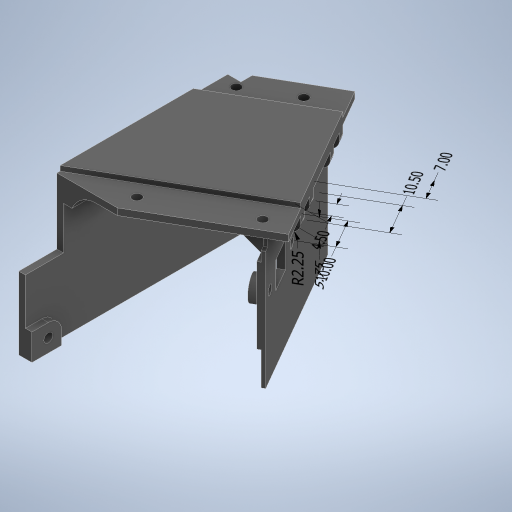
# Autodesk Inventor part: flame_side_right
Saved by Autodesk Inventor 2024.1 (Build 281209000, 209)
## iProperties
Created: 2025-03-06
Part Number: flame_side_right
Material: 一般
Document SubType Name: Modeling
Designer: hibik
Density: 1 g/cm^3
Appearance: 既定
Author: hibik
Autodesk Inventor part; units mm, degrees
ref_plane "YZ Plane" through (0, 0, 0) normal (1, 0, 0) x (0, 1, 0)
ref_plane "XZ Plane" through (0, 0, 0) normal (0, 1, 0) x (-1, 0, 0)
ref_plane "XY Plane" through (0, 0, 0) normal (0, 0, 1) x (1, 0, 0)
sketch "スケッチ1" plane through (0, 0, 0) normal (0, 1, 0) x (-1, 0, 0)
  line L0 (0, 0) -> (-75, 129.9038)
  line L1 (0, 0) -> (9.1573, 5.287) construction
  line L2 (-46.25, 80.1073) -> (0, 106.8098)
  line L3 (-28.75, 49.7965) -> (0, 66.3953)
  line L4 (-37.5, 64.9519) -> (-18.3005, 76.0367) construction
  line L5 (25.9887, 0) -> (-91.8315, 0) projected
  line L6 (0, 0) -> (0, 106.8098)
  line L7 (-51.25, 88.7676) -> (0, 118.3568)
  line L8 (0, 118.3568) -> (0, 106.8098)
  line L9 (-23.75, 41.1362) -> (0, 54.8483)
  dimension "d0" = 150
  dimension "d1" = 60
  dimension "d2" = 57.5
  dimension "d5" = 10
  constraints: 18 end point, 6 point on line, 4 perpendicular, 2 vertical, 1 midpoint, 1 parallel, 2 other
  measures "d0" distance from line of L0.end L1
  measures "d1" angle of L0 L5
  measures "d2" distance between parallel lines of L1 L3
  measures "d5" distance between parallel lines of L3 L9
extrude "押し出し1" add sketch "スケッチ1" along normal blind 1.5 contours L0 L2 L6 L3
extrude "押し出し2" add sketch "スケッチ1" against normal blind 2 contours L0 L3 L6 L9 | L0 L2 L6 L3 | L0 L7 L8 L2
sketch "スケッチ2" plane through (0, 1.5, 66.3953) normal (-1, 0, 0) x (0, 0, 1)
  line L0 (-22.0385, -1.5) -> (52.9615, -1.5)
  line L1 (52.9615, -1.5) -> (52.9615, -43.5)
  line L2 (52.9615, -43.5) -> (-22.0385, -43.5)
  line L3 (-22.0385, -43.5) -> (-22.0385, -1.5)
  line L4 (40.4145, -1.5) -> (51.9615, -1.5) projected
  line L5 (-22.0385, -11.5) -> (52.9615, -11.5)
  line L6 (51.9615, -3.5) -> (-11.547, -3.5) projected
  line L7 (51.9615, -1.5) -> (51.9615, -3.5) projected
  point P0 (-66.3953, -1.5)
  point P1 (20.2073, -3.5)
  point P2 (15.4615, -11.5)
  dimension "d8" = 75
  dimension "d9" = 32
  dimension "d12" = 10
  dimension "d23" = 1
  constraints: 10 end point, 2 midpoint, 2 parallel, 2 perpendicular, 2 point on line, 1 collinear, 1 horizontal
  measures "d8" distance of L0.start L0.end
  measures "d9" distance between parallel lines of L2 L5
  measures "d12" distance between parallel lines of L0 L5
  measures "d23" distance between parallel lines of L7 L1
extrude "押し出し3" add sketch "スケッチ2" against normal blind 2
sketch "スケッチ3" plane through (2, 1.5, 66.3953) normal (1, 0, 0) x (0, 0, -1)
  circle A0 centre (-47.9615, -12.5) radius 4
  circle A1 centre (17.0385, -12.5) radius 4
  line L0 (-52.9615, -43.5) -> (22.0385, -43.5) projected
  line L1 (-52.9615, -8.5) -> (22.0385, -8.5)
  line L2 (22.0385, -43.5) -> (22.0385, -1.5) projected
  line L3 (-51.9615, -8.5) -> (-51.9615, -18.5112) construction
  line L4 (-52.9615, -8.5) -> (-43.9615, -8.5)
  line L5 (-43.9615, -8.5) -> (-43.9615, -16.5)
  line L6 (-43.9615, -16.5) -> (-52.9615, -16.5)
  line L7 (-52.9615, -16.5) -> (-52.9615, -8.5)
  line L8 (22.0385, -8.5) -> (13.0385, -8.5)
  line L9 (13.0385, -8.5) -> (13.0385, -16.5)
  line L10 (13.0385, -16.5) -> (22.0385, -16.5)
  line L11 (22.0385, -16.5) -> (22.0385, -8.5)
  line L12 (22.0385, -1.5) -> (0, -1.5) projected
  line L13 (0, 0) -> (-40.4145, 0) projected
  line L14 (-40.4145, -1.5) -> (0, -1.5) projected
  line L15 (-40.4145, -1.5) -> (-40.4145, 0) projected
  line L16 (0, -1.5) -> (0, 0) projected
  line L17 (-40.4145, -1.5) -> (0, -1.5)
  line L18 (-52.9615, -1.5) -> (-52.9615, -43.5) projected
  line L19 (-40.4145, -1.5) -> (-52.9615, -1.5) projected
  line L20 (-52.9615, -35.5) -> (22.0385, -35.5)
  circle A2 centre (-47.9615, -39.5) radius 4
  circle A3 centre (17.0385, -39.5) radius 4
  line L21 (-43.9615, -39.5) -> (-43.9615, -43.5)
  line L22 (13.0385, -39.5) -> (13.0385, -43.5)
  point P0 (66.3953, -1.5)
  point P1 (13.0385, -12.5)
  point P2 (17.0385, -16.5)
  point P3 (22.0385, -16.5)
  point P4 (-47.9615, -16.5)
  point P5 (-43.9615, -12.5)
  point P6 (-47.9615, -8.5)
  point P7 (-47.9615, -35.5)
  point P8 (17.0385, -35.5)
  dimension "d13" = 8
  dimension "d14" = 35
  dimension "d15" = 65
  dimension "d24" = 1
  constraints: 28 end point, 7 horizontal, 7 tangent, 6 point on line, 5 perpendicular, 4 parallel, 3 vertical, 2 centre point, 2 vertical alignment, 1 collinear, 1 equal radius, 7 other
  measures "d13" diameter of A0
  measures "d14" distance between parallel lines of L0 L1
  measures "d15" distance of A1.centre A0.centre
  measures "d24" distance between parallel lines of L18 L3
extrude "押し出し4" add sketch "スケッチ3" along normal blind 2 contours A0 | A0 L1 L5 | A0 L6 L7 L1 | L1 L18 L19 L14 L12 L2 | L1 A1 L9 | L20 A2 L0 L18 | L1 L2 L10 A1 | A1 | A2 | A2 L21 L0 | L20 L2 L0 A3 | A3 | A3 L0 L22
sketch "スケッチ4" plane through (4, 1.5, 66.3953) normal (1, 0, 0) x (0, 0, -1)
  arc A0 (-47.9615, -16.5) -> (-43.9615, -12.5) centre (-47.9615, -12.5) ccw projected
  arc A1 (13.0385, -12.5) -> (17.0385, -16.5) centre (17.0385, -12.5) ccw projected
  circle A2 centre (-47.9615, -12.5) radius 1.35
  circle A3 centre (17.0385, -12.5) radius 1.35
  circle A4 centre (17.0385, -39.5) radius 1.35
  circle A5 centre (-47.9615, -39.5) radius 1.35
  arc A6 (17.0385, -35.5) -> (13.0385, -39.5) centre (17.0385, -39.5) ccw projected
  arc A7 (-43.9615, -39.5) -> (-47.9615, -35.5) centre (-47.9615, -39.5) ccw projected
  point P0 (66.3953, -1.5)
  dimension "d19" = 2.7
  dimension "d20" = 2.7
  constraints: 4 centre point, 2 coincident, 2 concentric, 2 equal radius
  measures "d19" diameter of A2
  measures "d20" diameter of A3
extrude "押し出し5" cut sketch "スケッチ4" against normal through all
sketch "スケッチ5" plane through (0, -2, 0) normal (0, -1, 0) x (1, 0, 0)
  line L0 (31.6173, 108.7628) -> (-5, 108.7628) construction
  line L1 (51.25, 88.7676) -> (4, 116.0474) projected
  line L2 (0, 44.3568) -> (0, 119.3568) projected
  line L3 (18.3494, 107.7628) -> (0, 107.7628)
  line L4 (4, 116.0474) -> (4, 119.3568) projected
  line L5 (0, 119.3568) -> (4, 119.3568) projected
  point P0 (0, 0)
  point P1 (0, 106.8098)
  dimension "d25" = 1
  constraints: 2 end point, 2 point on line, 1 parallel
  measures "d25" distance between parallel lines of L0 L3
extrude "押し出し6" cut sketch "スケッチ5" along normal mid plane 10
fillet "フィレット1" radius 8 1 edges at (4, -2, 80.1508)
sketch "スケッチ6" plane through (0, 0, 0) normal (0, 1, 0) x (1, 0, 0)
  circle A0 centre (17.5897, -50.4663) radius 1.6 construction
  circle A1 centre (4.5994, -57.9663) radius 1.6 construction
  circle A2 centre (43.3666, -88.7131) radius 1.6 construction
  circle A3 centre (18.4391, -101.9375) radius 1.6 construction
  circle A4 centre (17.5897, -50.4663) radius 1.35
  circle A5 centre (4.5994, -57.9663) radius 1.35
  circle A6 centre (18.4391, -101.9375) radius 1.35
  circle A7 centre (43.3666, -88.7131) radius 1.35
  point P0 (0, 0)
  dimension "d29" = 2.7
  constraints: 4 centre point, 4 coincident, 3 equal radius
  measures "d29" diameter of A4
extrude "押し出し7" cut sketch "スケッチ6" against normal through all
ref_plane "作業平面2" through (3.75, 0, 72.8905) normal (-0.5, 0, -0.8660254) x (-0.8660254, 0, 0.5)
ref_plane "作業平面1" through (8.75, 0, 81.5507) normal (-0.5, 0, -0.8660254) x (-0.8660254, 0, 0.5)
sketch "スケッチ7" plane through (3.75, 0, 72.8905) normal (-0.5, 0, -0.8660254) x (-0.8660254, 0, 0.5)
  circle A0 centre (-30.9476, -4.25) radius 2.25
  circle A1 centre (-30.9476, -4.25) radius 1
  line L0 (-33.1976, -2) -> (4.7927, -2) projected
  line L1 (-33.1976, 0) -> (-33.1976, -2) projected
  line L2 (-33.1976, -2) -> (-33.1976, -4.25)
  line L3 (-28.6976, -4.25) -> (-28.6976, -2)
  point P0 (-30.9476, -2)
  dimension "d33" = 2
  dimension "d34" = 4.5
  constraints: 4 end point, 3 tangent, 2 centre point, 2 point on circle, 1 coincident, 1 parallel, 1 point on line, 1 vertical
  measures "d33" diameter of A1
  measures "d34" diameter of A0
extrude "押し出し8" add sketch "スケッチ7" against normal blind 3
sketch "スケッチ8" plane through (0, 0, 66.3953) normal (-0.5, 0, -0.8660254) x (-0.8660254, 0, 0.5)
  arc A0 (-33.1976, -4.25) -> (-28.6976, -4.25) centre (-30.9476, -4.25) ccw projected
  circle A1 centre (-30.9476, -4.25) radius 1 projected
  line L0 (-28.6976, -4.25) -> (-28.6976, -2) projected
  line L1 (-33.1976, -2) -> (-28.6976, -2) projected
  line L2 (-33.1976, -2) -> (-33.1976, -4.25) projected
  point P0 (-33.1976, 0)
extrude "押し出し9" add sketch "スケッチ8" against normal blind 3
mirror "ミラー1" about plane through (8.75, 0, 81.5507) normal (-0.5, 0, -0.8660254) of "押し出し9", "押し出し8"
sketch "スケッチ9" plane through (0, 1.5, 66.3953) normal (-1, 0, 0) x (0, 0, 1)
  line L0 (-22.0385, -8.5) -> (-10.4445, -8.5)
  line L1 (-10.4445, -8.5) -> (-10.4445, -21.5)
  line L2 (-10.4445, -21.5) -> (-22.0385, -21.5)
  line L3 (-22.0385, -21.5) -> (-22.0385, -8.5)
  line L4 (41.3675, -8.5) -> (52.9615, -8.5)
  line L5 (52.9615, -8.5) -> (52.9615, -21.5)
  line L6 (52.9615, -21.5) -> (41.3675, -21.5)
  line L7 (41.3675, -21.5) -> (41.3675, -8.5)
  line L8 (52.9615, -43.5) -> (52.9615, -8.5) projected
  line L9 (52.9615, -8.5) -> (41.3675, -8.5) projected
  line L10 (-22.0385, -1.5) -> (-22.0385, -43.5) projected
  line L11 (41.3675, -8.5) -> (41.3675, -1.5) projected
  line L12 (-10.4445, -8.5) -> (-10.4445, -1.5)
  line L13 (-22.0385, -1.5) -> (0, -1.5) projected
  point P0 (-66.3953, -1.5)
  dimension "d60" = 0
  dimension "d63" = 13
  constraints: 18 end point, 4 parallel, 3 collinear, 2 equal length, 2 horizontal, 2 perpendicular, 2 point on line, 1 vertical
  measures "d60" distance between parallel lines of L9 L4
  measures "d63" distance between parallel lines of L6 L4
extrude "押し出し10" cut sketch "スケッチ9" against normal up to surface (4 mm away)
sketch "スケッチ10" plane through (0, -2, 0) normal (0, -1, 0) x (1, 0, 0)
  line L0 (4, 55.9508) -> (0, 55.9508) projected
  line L1 (0, 55.9508) -> (0, 66.3953) projected
  line L2 (28.75, 49.7965) -> (0, 66.3953) projected
  line L3 (28.75, 49.7965) -> (23.75, 41.1362) projected
  line L4 (23.75, 41.1362) -> (4, 52.5389) projected
  line L5 (4, 52.5389) -> (4, 55.9508) projected
  circle A0 centre (4.5994, 57.9663) radius 1.35 projected
  circle A1 centre (17.5897, 50.4663) radius 1.35 projected
  line L6 (0, 44.3568) -> (0, 119.3568) projected
  line L7 (0, 44.3568) -> (4, 44.3568) projected
  line L8 (4, 53.3568) -> (4, 44.3568) projected
  line L9 (2, 53.3568) -> (4, 53.3568) projected
  line L10 (2, 110.3568) -> (2, 53.3568) projected
  line L11 (2, 110.3568) -> (4, 110.3568) projected
  line L12 (4, 119.3568) -> (4, 110.3568) projected
  line L13 (0, 119.3568) -> (4, 119.3568) projected
  line L14 (4, 55.9508) -> (18.0903, 55.9508)
  point P0 (0, 0)
  constraints: 2 end point, 1 horizontal, 1 point on line
extrude "押し出し11" cut sketch "スケッチ10" along normal through all contours L14 L2 L3 L4 L5
sketch "スケッチ11" plane through (0, -2, 0) normal (0, -1, 0) x (1, 0, 0)
  line L0 (46.0538, 91.7676) -> (18.5538, 44.1362)
  line L1 (18.5538, 44.1362) -> (16.8218, 45.1362)
  line L2 (16.8218, 45.1362) -> (44.3218, 92.7676)
  line L3 (44.3218, 92.7676) -> (46.0538, 91.7676)
  line L4 (34, 58.8897) -> (41, 71.0141) projected
  line L5 (51.25, 88.7676) -> (18.3494, 107.7628) projected
  line L6 (4, 52.5389) -> (23.75, 41.1362) projected
  point P0 (0, 0)
  dimension "d66" = 2
  dimension "d68" = 6
  constraints: 8 end point, 3 parallel, 2 collinear, 1 perpendicular
  measures "d66" distance between parallel lines of L2 L0
  measures "d68" distance between parallel lines of L4 L0
extrude "押し出し12" add sketch "スケッチ11" along normal blind 22
sketch "スケッチ14" plane through (16.8218, -24, 45.1362) normal (-0.8660254, 0, 0.5) x (0.5, 0, 0.8660254)
  line L0 (51.6296, 22) -> (55, 22) projected
  line L1 (51.6296, 22) -> (50.3927, 22) projected
  line L2 (0, 22) -> (50.3927, 22) projected
  line L3 (0, 22) -> (0, 0) projected
  line L4 (55, 0) -> (0, 0) projected
  line L5 (55, 22) -> (55, 0) projected
  circle A0 centre (48, 3.5) radius 3.5
  circle A1 centre (30, 3.5) radius 3.5
  circle A2 centre (48, 3.5) radius 1.35
  circle A3 centre (30, 3.5) radius 1.35
  line L6 (39, 8.3219) -> (39, 1.6295) construction
  point P0 (-47.5, 24)
  dimension "d84" = 18
  dimension "d85" = 7
  dimension "d86" = 2.7
  dimension "d98" = 7
  constraints: 4 centre point, 2 end point, 1 coincident, 1 tangent, 1 vertical, 2 other
  measures "d84" distance of A0.centre A1.centre
  measures "d85" diameter of A1
  measures "d86" diameter of A2
  measures "d98" distance from line of L5 A0.centre
extrude "押し出し16" add sketch "スケッチ14" along normal blind 2 contours A1 | A0
extrude "押し出し17" cut sketch "スケッチ14" against normal through all contours A2 | A3
sketch "スケッチ15" plane through (46.0538, -24, 91.7676) normal (0.8660254, 0, -0.5) x (-0.5, 0, -0.8660254)
  line L0 (12.8975, 4.0421) -> (15.8975, 4.0421) construction
  line L1 (15.8975, 4.0421) -> (15.8975, 1.0421) construction
  line L2 (11.8975, 8.0843) -> (19.8975, 8.0843)
  line L3 (19.8975, 8.0843) -> (19.8975, 0)
  line L4 (19.8975, 0) -> (11.8975, 0)
  line L5 (11.8975, 0) -> (11.8975, 8.0843)
  line L6 (55, 0) -> (0, 0) projected
  line L7 (12.8975, 6.7421) -> (12.8975, 1.3421)
  line L8 (13.1975, 1.0421) -> (18.5975, 1.0421)
  point P0 (102.5, 24)
  dimension "d99" = 1
  constraints: 16 end point, 2 horizontal, 2 midpoint, 2 parallel, 2 perpendicular, 1 collinear, 1 vertical, 6 other
  measures "d99" distance between parallel lines of L5 L7
extrude "押し出し18" cut sketch "スケッチ15" against normal up to surface (2 mm away)
sketch "スケッチ16" plane through (0, 0, 0) normal (0, 1, 0) x (1, 0, 0)
  circle A0 centre (43.3666, -88.7131) radius 1.35 projected
  point P0 (0, 0)
extrude "押し出し19" cut sketch "スケッチ16" against normal blind 8
sketch "スケッチ17" plane through (46.0538, -24, 91.7676) normal (0.8660254, 0, -0.5) x (-0.5, 0, -0.8660254)
  circle A0 centre (7, 3.5) radius 3.5 projected
  line L0 (3.5, 3.5) -> (3.5, 22)
  line L1 (3.3704, 22) -> (0, 22) projected
  line L2 (0, 22) -> (2.9015, 22) projected
  line L3 (4.6073, 22) -> (3.3704, 22) projected
  line L4 (0, 22) -> (0, 0) projected
  line L5 (11.8975, 0) -> (0, 0) projected
  line L6 (3.5, 3.5) -> (3.5, 0)
  point P0 (102.5, 24)
  constraints: 4 end point, 2 perpendicular, 2 point on line, 1 horizontal alignment, 1 vertical, 1 other
extrude "押し出し20" cut sketch "スケッチ17" against normal up to surface (2 mm away) contours L6 L5 L4 L1 L3 L0
sketch "スケッチ18" plane through (0, -24, 0) normal (0, -1, 0) x (1, 0, 0)
  line L0 (36.1051, 74.5359) -> (34.3731, 75.5359) projected
  line L1 (34.3731, 75.5359) -> (31.8218, 71.117) projected
  line L2 (31.8218, 71.117) -> (16.8218, 45.1362) projected
  line L3 (16.8218, 45.1362) -> (18.5538, 44.1362) projected
  line L4 (18.5538, 44.1362) -> (36.1051, 74.5359) projected
  line L5 (44.3038, 88.7365) -> (42.5718, 89.7365) projected
  line L6 (42.5718, 89.7365) -> (40.8218, 86.7054) projected
  line L7 (40.8218, 86.7054) -> (38.3731, 82.4641) projected
  line L8 (38.3731, 82.4641) -> (40.1051, 81.4641) projected
  line L9 (40.1051, 81.4641) -> (44.3038, 88.7365) projected
  line L10 (40.1051, 81.4641) -> (36.1051, 74.5359)
  line L11 (34.3731, 75.5359) -> (38.3731, 82.4641)
  point P0 (0, 0)
  constraints: 4 end point, 1 collinear, 1 parallel
extrude "押し出し21" add sketch "スケッチ18" along normal blind 20
ref_plane "作業平面3" through (47.75, -2, 82.7054) normal (0.5, 0, 0.8660254) x (0.8660254, 0, -0.5)
sketch "スケッチ19" plane through (47.75, -2, 82.7054) normal (0.5, 0, 0.8660254) x (0.8660254, 0, -0.5)
  line L0 (-8, -6) -> (-8, 0) projected
  line L1 (-22.8053, 0) -> (-8, 0) projected
  line L2 (-22.8053, 0) -> (-22.8053, 2) projected
  line L3 (0, 2) -> (-22.8053, 2) projected
  line L4 (0, 2) -> (0, 0) projected
  line L5 (-6, 0) -> (0, 0) projected
  line L6 (-6, 0) -> (-6, -42) projected
  line L7 (-8, -42) -> (-6, -42) projected
  line L8 (-8, 0) -> (-8, -42) projected
  line L9 (-8, -9) -> (-17, 0)
  point P0 (0, 2)
  point P1 (-8, 0)
  dimension "d105" = 9
  dimension "d106" = 9
  constraints: 2 end point, 2 point on line
  measures "d105" distance of L0.end L9.start
  measures "d106" distance of L0.end L9.end
extrude "押し出し22" add sketch "スケッチ19" against normal blind 23 contours L8 L9 L1 L0
sketch "スケッチ20" plane through (42.0181, -8, 88.7775) normal (-0.8660254, 0, 0.5) x (0.5, 0, 0.8660254)
  line L0 (-2.3927, 6) -> (-2.3927, -3) projected
  line L1 (-2.3927, -3) -> (-25.3927, -3) projected
  line L2 (-25.3927, -3) -> (-25.3927, 6) projected
  line L3 (-50.3927, 6) -> (-25.3927, 6) projected
  line L4 (-50.3927, 6) -> (-50.3927, -36) projected
  line L5 (1.1073, -36) -> (-50.3927, -36) projected
  line L6 (1.1073, -36) -> (1.1073, -12.5) projected
  circle A0 centre (-2.3927, -12.5) radius 3.5 projected
  line L7 (1.1073, -12.5) -> (1.1073, 0) projected
  line L8 (1.1073, 0) -> (0, 0) projected
  line L9 (0, 0) -> (0, 6) projected
  line L10 (-2.3927, 6) -> (0, 6) projected
  circle A1 centre (-20.3927, -12.5) radius 3.5 projected
  line L11 (-15.2901, -16) -> (-15.2901, -7.9157) projected
  line L12 (-15.2901, -7.9157) -> (-7.2901, -7.9157) projected
  line L13 (-7.2901, -7.9157) -> (-7.2901, -16) projected
  line L14 (-7.2901, -16) -> (-15.2901, -16) projected
  line L15 (1.1073, -3) -> (-25.3927, -3)
  line L16 (-25.3927, -3) -> (-25.3927, -26)
  line L17 (-25.3927, -26) -> (1.1073, -26)
  line L18 (1.1073, -26) -> (1.1073, -3)
  point P0 (-97.8927, 8)
  point P1 (1.1073, -26)
  dimension "d110" = 23
  constraints: 8 end point, 2 parallel, 2 point on line, 1 collinear, 1 horizontal, 1 horizontal alignment, 1 perpendicular
  measures "d110" distance between parallel lines of L17 L15
extrude "押し出し23" cut sketch "スケッチ20" against normal blind 1 contours L10 L9 L8 L7 L15 L0 | L16 L17 L6 L5 L4 L3 L2
equation "\"d106\" = d105"
